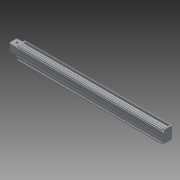
# Autodesk Inventor part: GL20N41420CSW' Body2
Saved by Autodesk Inventor 2011 SP1 (Build 150282100, 282)
## iProperties
Created: 2013-11-12
Part Number: GL20N41420CSW' Body2
Catalog Web Link: www.cadenas.de
Description: Type GL-N-body2-
Vendor: THK
Document SubType Name: Modeling
Designer: PARTuser1
Manufacturer: THK
Density: 1 g/cm^3
Category: PARTsolutions
Company: THK
Title: GL20N41420CSW' Body2
Author: Cadenas PARTsolutions
PSOL_IDENT_0: {$CADENAS_DATA\23d-libs\thk\actuator\type_gl_n\type_gl_n_f_na_1.prj},213 {VTYP=3D},{NB=GL20N41420CSW
PSOL_IDENT_1: ' Body2},{LINA=GL20N41420CSW' Body2},{NN=Type GL-N-body2},{DATE=29.11.2012 11:43:39},{GEOMDATE=29.11
PSOL_IDENT_2: .2012 11:43:00},{VERSION=},{LINEID=40},{LINESUBID=-1},{WBVAR=L,C,LM,BSE,BSM,LML,BSL}  {NB=GL20N41420
PSOL_IDENT_3: CSW' Body2},{LINA=GL20N41420CSW' Body2},{KT=DUMMY},{IDNR=},{MN=GL20N},{L=1420},{C=C},{LX=460,580,700
PSOL_IDENT_4: ,820,1060,1240,1420,1600,1780,1960,2200,2320,2500,3000},{LM=SW},{VER=4},{DS=Belt kit},{BSE=},{R=25.0
PSOL_IDENT_5: 00},{NDM=2.000},{PCD=0.000},{BSM=},{BSE1='','None'},{SD=39},{SD1=27},{TL=180.000},{B=65.000},{TL1=21
PSOL_IDENT_6: 0.000},{B1=70.000},{DS1=Ex},{LML='},{BSL=},{BSL1='','None'},{N=9},{N1=6},{N2=8.000},{N3=6},{BSM1='',
PSOL_IDENT_7: 'None'}
CNS_NN: Type GL-N-body2
CNS_NB: GL20N41420CSW' Body2
CNS_NBSYN: $MN.$VER.$L.$C.$BSE.$BSM.$LM.$LML.$BSL. Body2
CNS_LINA: GL20N41420CSW' Body2
CNS_MN: GL20N
CNS_L: 1420
CNS_C: Yes
CNS_LX: 460,580,700,820,1060,1240,1420,1600,1780,1960,2200,2320,2500,3000
CNS_LM: SSR-XW (L-type table)
CNS_VER: 4
CNS_DS: Belt kit
CNS_R: 25.000
CNS_NDM: 2.000
CNS_PCD: 0.000
CNS_BSE1: '','None'
CNS_SD: 39
CNS_SD1: 27
CNS_TL: 180.000
CNS_B: 65.000
CNS_TL1: 210.000
CNS_B1: 70.000
CNS_DS1: Ex
CNS_LML: No mark:Not provided with QZ
CNS_BSL1: '','None'
CNS_N: 9.000
CNS_N1: 6.000
CNS_N2: 8.000
CNS_N3: 6.000
CNS_BSM1: '','None'
SUPPLIER: THK
ARTICLENO: GL20N41420CSW' Body2
BOMINFO: GL20N41420CSW' Body2
CREATOR: CADENAS GmbH
Autodesk Inventor part; units mm, degrees
sketch "Sketch_1" plane through (0, 0, 0) normal (1, 0, 0) x (0, 1, 0)
  line L0 (39, 65) -> (37, 65)
  line L1 (37, 65) -> (37, 64)
  line L2 (37, 64) -> (33.72, 64)
  arc A0 (33.72, 64) -> (33.25, 63.53) centre (33.72, 63.53) ccw
  line L3 (33.25, 63.53) -> (33.25, 62.97)
  arc A1 (33.25, 62.97) -> (33.72, 62.5) centre (33.72, 62.97) ccw
  line L4 (33.72, 62.5) -> (33.93, 62.5)
  arc A2 (34.4, 62.03) -> (33.93, 62.5) centre (33.93, 62.03) ccw
  line L5 (34.4, 62.03) -> (34.4, 60.47)
  arc A3 (33.93, 60) -> (34.4, 60.47) centre (33.93, 60.47) ccw
  line L6 (33.93, 60) -> (33.7, 60)
  arc A4 (33.7, 60) -> (33.5, 59.8) centre (33.7, 59.8) ccw
  line L7 (33.5, 59.8) -> (33.5, 59.7)
  arc A5 (33.3, 59.5) -> (33.5, 59.7) centre (33.3, 59.7) ccw
  line L8 (33.3, 59.5) -> (29.7, 59.5)
  arc A6 (29.5, 59.7) -> (29.7, 59.5) centre (29.7, 59.7) ccw
  line L9 (29.5, 59.7) -> (29.5, 59.8)
  arc A7 (29.5, 59.8) -> (29.3, 60) centre (29.3, 59.8) ccw
  line L10 (29.3, 60) -> (29.07, 60)
  arc A8 (28.6, 60.47) -> (29.07, 60) centre (29.07, 60.47) ccw
  line L11 (28.6, 60.47) -> (28.6, 62.03)
  arc A9 (29.07, 62.5) -> (28.6, 62.03) centre (29.07, 62.03) ccw
  line L12 (29.07, 62.5) -> (29.28, 62.5)
  arc A10 (29.28, 62.5) -> (29.75, 62.97) centre (29.28, 62.97) ccw
  line L13 (29.75, 62.97) -> (29.75, 63.7)
  arc A11 (29.75, 63.7) -> (29.45, 64) centre (29.45, 63.7) ccw
  line L14 (29.45, 64) -> (26, 64)
  line L15 (26, 64) -> (26, 65)
  line L16 (26, 65) -> (12.3, 65)
  arc A12 (12.3, 65) -> (12, 64.7) centre (12.3, 64.7) ccw
  line L17 (12, 64.7) -> (12, 60.8)
  arc A13 (11.7, 60.5) -> (12, 60.8) centre (11.7, 60.8) ccw
  line L18 (11.7, 60.5) -> (6.3, 60.5)
  arc A14 (6, 60.8) -> (6.3, 60.5) centre (6.3, 60.8) ccw
  line L19 (6, 60.8) -> (6, 64.7)
  arc A15 (6, 64.7) -> (5.7, 65) centre (5.7, 64.7) ccw
  line L20 (5.7, 65) -> (3.14, 65)
  arc A16 (3.14, 65) -> (0, 61.86) centre (3.14, 61.86) ccw
  line L21 (0, 61.86) -> (0, 53.47)
  arc A17 (0, 53.47) -> (0.47, 53) centre (0.47, 53.47) ccw
  line L22 (0.47, 53) -> (3.53, 53)
  arc A18 (3.53, 53) -> (4, 53.47) centre (3.53, 53.47) ccw
  line L23 (4, 53.47) -> (4, 55.03)
  arc A19 (4.47, 55.5) -> (4, 55.03) centre (4.47, 55.03) ccw
  line L24 (4.47, 55.5) -> (8.53, 55.5)
  arc A20 (9, 55.03) -> (8.53, 55.5) centre (8.53, 55.03) ccw
  line L25 (9, 55.03) -> (9, 53.7)
  arc A21 (9, 53.7) -> (9.2, 53.5) centre (9.2, 53.7) ccw
  line L26 (9.2, 53.5) -> (9.53, 53.5)
  arc A22 (10, 53.03) -> (9.53, 53.5) centre (9.53, 53.03) ccw
  line L27 (10, 53.03) -> (10, 46.97)
  arc A23 (9.53, 46.5) -> (10, 46.97) centre (9.53, 46.97) ccw
  line L28 (9.53, 46.5) -> (9.2, 46.5)
  arc A24 (9.2, 46.5) -> (9, 46.3) centre (9.2, 46.3) ccw
  line L29 (9, 46.3) -> (9, 44.97)
  arc A25 (8.53, 44.5) -> (9, 44.97) centre (8.53, 44.97) ccw
  line L30 (8.53, 44.5) -> (4.47, 44.5)
  arc A26 (4, 44.97) -> (4.47, 44.5) centre (4.47, 44.97) ccw
  line L31 (4, 44.97) -> (4, 46.53)
  arc A27 (4, 46.53) -> (3.53, 47) centre (3.53, 46.53) ccw
  line L32 (3.53, 47) -> (0.47, 47)
  arc A28 (0.47, 47) -> (0, 46.53) centre (0.47, 46.53) ccw
  line L33 (0, 46.53) -> (0, 25)
  line L34 (0, 25) -> (1.3137, 18.3899)
  arc A29 (1.3469, 17.8569) -> (1.3137, 18.3899) centre (-0.6479, 18) ccw
  arc A30 (1.3469, 17.8569) -> (1.3469, -17.8569) centre (250.2071, 0) ccw
  arc A31 (1.3137, -18.3899) -> (1.3469, -17.8569) centre (-0.6479, -18) ccw
  line L35 (1.3137, -18.3899) -> (0, -25)
  line L36 (0, -25) -> (0, -46.53)
  arc A32 (0, -46.53) -> (0.47, -47) centre (0.47, -46.53) ccw
  line L37 (0.47, -47) -> (3.53, -47)
  arc A33 (3.53, -47) -> (4, -46.53) centre (3.53, -46.53) ccw
  line L38 (4, -46.53) -> (4, -44.97)
  arc A34 (4.47, -44.5) -> (4, -44.97) centre (4.47, -44.97) ccw
  line L39 (4.47, -44.5) -> (8.53, -44.5)
  arc A35 (9, -44.97) -> (8.53, -44.5) centre (8.53, -44.97) ccw
  line L40 (9, -44.97) -> (9, -46.3)
  arc A36 (9, -46.3) -> (9.2, -46.5) centre (9.2, -46.3) ccw
  line L41 (9.2, -46.5) -> (9.53, -46.5)
  arc A37 (10, -46.97) -> (9.53, -46.5) centre (9.53, -46.97) ccw
  line L42 (10, -46.97) -> (10, -53.03)
  arc A38 (9.53, -53.5) -> (10, -53.03) centre (9.53, -53.03) ccw
  line L43 (9.53, -53.5) -> (9.2, -53.5)
  arc A39 (9.2, -53.5) -> (9, -53.7) centre (9.2, -53.7) ccw
  line L44 (9, -53.7) -> (9, -55.03)
  arc A40 (8.53, -55.5) -> (9, -55.03) centre (8.53, -55.03) ccw
  line L45 (8.53, -55.5) -> (4.47, -55.5)
  arc A41 (4, -55.03) -> (4.47, -55.5) centre (4.47, -55.03) ccw
  line L46 (4, -55.03) -> (4, -53.47)
  arc A42 (4, -53.47) -> (3.53, -53) centre (3.53, -53.47) ccw
  line L47 (3.53, -53) -> (0.47, -53)
  arc A43 (0.47, -53) -> (0, -53.47) centre (0.47, -53.47) ccw
  line L48 (0, -53.47) -> (0, -61.86)
  arc A44 (0, -61.86) -> (3.14, -65) centre (3.14, -61.86) ccw
  line L49 (3.14, -65) -> (5.7, -65)
  arc A45 (5.7, -65) -> (6, -64.7) centre (5.7, -64.7) ccw
  line L50 (6, -64.7) -> (6, -60.8)
  arc A46 (6.3, -60.5) -> (6, -60.8) centre (6.3, -60.8) ccw
  line L51 (6.3, -60.5) -> (11.7, -60.5)
  arc A47 (12, -60.8) -> (11.7, -60.5) centre (11.7, -60.8) ccw
  line L52 (12, -60.8) -> (12, -64.7)
  arc A48 (12, -64.7) -> (12.3, -65) centre (12.3, -64.7) ccw
  line L53 (12.3, -65) -> (26, -65)
  line L54 (26, -65) -> (26, -64)
  line L55 (26, -64) -> (29.45, -64)
  arc A49 (29.45, -64) -> (29.75, -63.7) centre (29.45, -63.7) ccw
  line L56 (29.75, -63.7) -> (29.75, -62.97)
  arc A50 (29.75, -62.97) -> (29.28, -62.5) centre (29.28, -62.97) ccw
  line L57 (29.28, -62.5) -> (29.07, -62.5)
  arc A51 (28.6, -62.03) -> (29.07, -62.5) centre (29.07, -62.03) ccw
  line L58 (28.6, -62.03) -> (28.6, -60.47)
  arc A52 (29.07, -60) -> (28.6, -60.47) centre (29.07, -60.47) ccw
  line L59 (29.07, -60) -> (29.3, -60)
  arc A53 (29.3, -60) -> (29.5, -59.8) centre (29.3, -59.8) ccw
  line L60 (29.5, -59.8) -> (29.5, -59.7)
  arc A54 (29.7, -59.5) -> (29.5, -59.7) centre (29.7, -59.7) ccw
  line L61 (29.7, -59.5) -> (33.3, -59.5)
  arc A55 (33.5, -59.7) -> (33.3, -59.5) centre (33.3, -59.7) ccw
  line L62 (33.5, -59.7) -> (33.5, -59.8)
  arc A56 (33.5, -59.8) -> (33.7, -60) centre (33.7, -59.8) ccw
  line L63 (33.7, -60) -> (33.93, -60)
  arc A57 (34.4, -60.47) -> (33.93, -60) centre (33.93, -60.47) ccw
  line L64 (34.4, -60.47) -> (34.4, -62.03)
  arc A58 (33.93, -62.5) -> (34.4, -62.03) centre (33.93, -62.03) ccw
  line L65 (33.93, -62.5) -> (33.72, -62.5)
  arc A59 (33.72, -62.5) -> (33.25, -62.97) centre (33.72, -62.97) ccw
  line L66 (33.25, -62.97) -> (33.25, -63.53)
  arc A60 (33.25, -63.53) -> (33.72, -64) centre (33.72, -63.53) ccw
  line L67 (33.72, -64) -> (37, -64)
  line L68 (37, -64) -> (37, -65)
  line L69 (37, -65) -> (39, -65)
  line L70 (39, -65) -> (39, -41)
  line L71 (39, -41) -> (43.5, -41)
  line L72 (43.5, -41) -> (43.5, -37)
  line L73 (43.5, -37) -> (21, -37)
  arc A61 (19, -35) -> (21, -37) centre (21, -35) ccw
  line L74 (19, -35) -> (19, 35)
  arc A62 (21, 37) -> (19, 35) centre (21, 35) ccw
  line L75 (21, 37) -> (43.5, 37)
  line L76 (43.5, 37) -> (43.5, 41)
  line L77 (43.5, 41) -> (39, 41)
  line L78 (39, 41) -> (39, 65)
  constraints: 158 end point, 126 point on circle, 63 centre point
extrude "Extrusion1" add sketch "Sketch_1" along normal blind 1420
sketch "Sketch_41" plane through (0, 0, 0) normal (1, 0, 0) x (0, 1, 0)
  line L0 (54.4, -41) -> (51.5, -41)
  line L1 (51.5, -41) -> (49.5, -43)
  line L2 (49.5, -43) -> (46, -43)
  line L3 (46, -43) -> (44, -41)
  line L4 (44, -41) -> (40, -41)
  line L5 (40, -41) -> (39, -42)
  line L6 (39, -42) -> (39, -60)
  line L7 (39, -60) -> (40, -61)
  line L8 (40, -61) -> (44, -61)
  line L9 (44, -61) -> (46, -59)
  line L10 (46, -59) -> (49.5, -59)
  line L11 (49.5, -59) -> (51.5, -61)
  line L12 (51.5, -61) -> (54.4, -61)
  line L13 (54.4, -61) -> (55.5, -59.9)
  line L14 (55.5, -59.9) -> (55.5, -42.1)
  line L15 (55.5, -42.1) -> (54.4, -41)
  constraints: 32 end point
extrude "Extrusion2" add sketch "Sketch_41" along normal blind 1420
sketch "Sketch_42" plane through (0, 0, 0) normal (1, 0, 0) x (0, 1, 0)
  line L0 (51.5, 61) -> (49.5, 59)
  line L1 (49.5, 59) -> (46, 59)
  line L2 (46, 59) -> (44, 61)
  line L3 (44, 61) -> (40, 61)
  line L4 (40, 61) -> (39, 60)
  line L5 (39, 60) -> (39, 42)
  line L6 (39, 42) -> (40, 41)
  line L7 (40, 41) -> (44, 41)
  line L8 (44, 41) -> (46, 43)
  line L9 (46, 43) -> (49.5, 43)
  line L10 (49.5, 43) -> (51.5, 41)
  line L11 (51.5, 41) -> (54.4, 41)
  line L12 (54.4, 41) -> (55.5, 42.1)
  line L13 (55.5, 42.1) -> (55.5, 59.9)
  line L14 (55.5, 59.9) -> (54.4, 61)
  line L15 (54.4, 61) -> (51.5, 61)
  constraints: 32 end point
extrude "Extrusion3" add sketch "Sketch_42" along normal blind 1420
sketch "Sketch_2" plane through (0, 0, 0) normal (1, 0, 0) x (0, 1, 0)
  line L0 (82, 60) -> (13, 60)
  line L1 (13, 60) -> (11, 58)
  line L2 (11, 58) -> (11, 45.64)
  arc A0 (7.86, 42.5) -> (11, 45.64) centre (7.86, 45.64) ccw
  line L3 (7.86, 42.5) -> (4, 42.5)
  line L4 (4, 42.5) -> (2, 40.5)
  line L5 (2, 40.5) -> (2, -40.5)
  line L6 (2, -40.5) -> (4, -42.5)
  line L7 (4, -42.5) -> (7.86, -42.5)
  arc A1 (11, -45.64) -> (7.86, -42.5) centre (7.86, -45.64) ccw
  line L8 (11, -45.64) -> (11, -58)
  line L9 (11, -58) -> (13, -60)
  line L10 (13, -60) -> (82, -60)
  line L11 (82, -60) -> (83, -59)
  line L12 (83, -59) -> (83, -50)
  line L13 (83, -50) -> (87, -50)
  line L14 (87, -50) -> (87, 50)
  line L15 (87, 50) -> (83, 50)
  line L16 (83, 50) -> (83, 59)
  line L17 (83, 59) -> (82, 60)
  constraints: 36 end point, 4 point on circle, 2 centre point
extrude "Extrusion4" add sketch "Sketch_2" against normal blind 12
sketch "Sketch_3" plane through (1420, 0, 0) normal (1, 0, 0) x (0, 0, -1)
  line L0 (-60, 82) -> (-60, 13)
  line L1 (-60, 13) -> (-58, 11)
  line L2 (-58, 11) -> (-45.64, 11)
  arc A0 (-42.5, 7.86) -> (-45.64, 11) centre (-45.64, 7.86) ccw
  line L3 (-42.5, 7.86) -> (-42.5, 4)
  line L4 (-42.5, 4) -> (-40.5, 2)
  line L5 (-40.5, 2) -> (40.5, 2)
  line L6 (40.5, 2) -> (42.5, 4)
  line L7 (42.5, 4) -> (42.5, 7.86)
  arc A1 (45.64, 11) -> (42.5, 7.86) centre (45.64, 7.86) ccw
  line L8 (45.64, 11) -> (58, 11)
  line L9 (58, 11) -> (60, 13)
  line L10 (60, 13) -> (60, 82)
  line L11 (60, 82) -> (59, 83)
  line L12 (59, 83) -> (50, 83)
  line L13 (50, 83) -> (50, 87)
  line L14 (50, 87) -> (-50, 87)
  line L15 (-50, 87) -> (-50, 83)
  line L16 (-50, 83) -> (-59, 83)
  line L17 (-59, 83) -> (-60, 82)
  constraints: 36 end point, 4 point on circle, 2 centre point
extrude "Extrusion5" add sketch "Sketch_3" along normal blind 12
sketch "Sketch_5" plane through (0, 0, 0) normal (1, 0, 0) x (0, 1, 0)
  line L0 (80.8094, -15) -> (76.1906, -15)
  line L1 (76.1906, -15) -> (73.8812, -19)
  line L2 (73.8812, -19) -> (76.1906, -23)
  line L3 (76.1906, -23) -> (80.8094, -23)
  line L4 (80.8094, -23) -> (83.1188, -19)
  line L5 (83.1188, -19) -> (80.8094, -15)
  constraints: 12 end point
extrude "Extrusion6" add sketch "Sketch_5" along normal blind 3.2
sketch "Sketch_6" plane through (0, 0, -19) normal (0, 0, 1) x (1, 0, 0)
  line L0 (15, 78.5) -> (3.2, 78.5)
  line L1 (3.2, 78.5) -> (3.2, 81)
  line L2 (3.2, 81) -> (6, 81)
  line L3 (6, 81) -> (6, 84.75)
  line L4 (6, 84.75) -> (15, 84.75)
  line L5 (15, 84.75) -> (15, 78.5)
  line L6 (15, 78.5) -> (3.2, 78.5)
  constraints: 14 end point
revolve "Revolution1" add sketch "Sketch_6" angle 360 about axis through (15, 78.5, -19) along (1, 0, 0)
sketch "Sketch8" plane through (1432, 0, 0) normal (1, 0, 0) x (0, 0, -1)
  point P0 (0, 78.5)
hole "Drilling 1" at (1432, 78.5, 0) direction (-1, 0, 0) diameter 4.134 depth 12 countersink diameter 5 countersink angle 90 thread size "M5x0.8" class "6H" standard "ISO Metric profile"
sketch "Sketch_7" plane through (1417.5, 0, 0) normal (1, 0, 0) x (0, 0, -1)
  line L0 (-29, 19) -> (29, 19)
  line L1 (29, 19) -> (29, 40.5)
  line L2 (29, 40.5) -> (-29, 40.5)
  line L3 (-29, 40.5) -> (-29, 19)
  constraints: 8 end point
extrude "Extrusion7" add sketch "Sketch_7" against normal blind 63
sketch "Sketch_8" plane through (0, 40.5, 0) normal (0, 1, 0) x (1, 0, 0)
  line L0 (1322, -29) -> (1403, -29)
  line L1 (1403, -29) -> (1403, 29)
  line L2 (1403, 29) -> (1322, 29)
  line L3 (1322, 29) -> (1322, 17)
  line L4 (1322, 17) -> (1357, 17)
  line L5 (1357, 17) -> (1357, -17)
  line L6 (1357, -17) -> (1322, -17)
  line L7 (1322, -17) -> (1322, -29)
  arc A0 (1362, -20.4) -> (1362, -25.6) centre (1362, -23) ccw
  line L8 (1362, -25.6) -> (1396, -25.6)
  arc A1 (1396, -25.6) -> (1396, -20.4) centre (1396, -23) ccw
  line L9 (1396, -20.4) -> (1362, -20.4)
  arc A2 (1362, 25.6) -> (1362, 20.4) centre (1362, 23) ccw
  line L10 (1362, 20.4) -> (1396, 20.4)
  arc A3 (1396, 20.4) -> (1396, 25.6) centre (1396, 23) ccw
  line L11 (1396, 25.6) -> (1362, 25.6)
  constraints: 24 end point, 8 point on circle, 4 centre point
extrude "Extrusion8" add sketch "Sketch_8" along normal blind 20
sketch "Sketch_9" plane through (0, 0, 0) normal (0, 0, 1) x (1, 0, 0)
  line L0 (-92, 84.3) -> (-92, 16.7)
  line L1 (-92, 16.7) -> (-87.8, 12.5)
  line L2 (-87.8, 12.5) -> (-12, 12.5)
  line L3 (-12, 12.5) -> (-12, 88.5)
  line L4 (-12, 88.5) -> (-87.8, 88.5)
  line L5 (-87.8, 88.5) -> (-92, 84.3)
  constraints: 12 end point
extrude "Extrusion9" add sketch "Sketch_9" along normal mid plane 72
sketch "Sketch_14" plane through (0, 25.5, 0) normal (0, 1, 0) x (1, 0, 0)
  arc A0 (-57, 25) -> (-57, -25) centre (-57, 0) ccw
  line L0 (-57, -25) -> (-12, -25)
  line L1 (-12, -25) -> (-12, -26)
  line L2 (-12, -26) -> (0, -26)
  line L3 (0, -26) -> (0, 24)
  line L4 (0, 24) -> (-12, 24)
  line L5 (-12, 24) -> (-12, 25)
  line L6 (-12, 25) -> (-57, 25)
  constraints: 14 end point, 2 point on circle, 1 centre point
extrude "Extrusion10" cut sketch "Sketch_14" along normal blind 50
sketch "Sketch_15" plane through (1332, 0, 0) normal (1, 0, 0) x (0, 0, -1)
  line L0 (31.15, 50.5) -> (-31.15, 50.5)
  line L1 (-31.15, 50.5) -> (-31.15, 55.5)
  line L2 (-31.15, 55.5) -> (-15.75, 55.5)
  line L3 (-15.75, 55.5) -> (-15.75, 66)
  line L4 (-15.75, 66) -> (-15.3, 66)
  line L5 (-15.3, 66) -> (-15.3, 73)
  line L6 (-15.3, 73) -> (-13.8, 73)
  line L7 (-13.8, 73) -> (-13.3, 69)
  line L8 (-13.3, 69) -> (13.3, 69)
  line L9 (13.3, 69) -> (13.8, 73)
  line L10 (13.8, 73) -> (15.3, 73)
  line L11 (15.3, 73) -> (15.3, 66)
  line L12 (15.3, 66) -> (15.75, 66)
  line L13 (15.75, 66) -> (15.75, 55.5)
  line L14 (15.75, 55.5) -> (31.15, 55.5)
  line L15 (31.15, 55.5) -> (31.15, 50.5)
  line L16 (31.15, 50.5) -> (-31.15, 50.5)
  constraints: 34 end point
revolve "Revolution2" add sketch "Sketch_15" angle 360 about axis through (1332, 50.5, -31.15) along (0, 0, -1)
sketch "Sketch14" plane through (0, 0, 36) normal (0, 0, 1) x (1, 0, 0)
  point P0 (-52, 50.5)
hole "Drilling 2" at (-52, 50.5, 36) direction (0, 0, -1) diameter 22 depth 4
sketch "Sketch15" plane through (0, 0, -36) normal (0, 0, -1) x (-1, 0, 0)
  point P0 (52, 50.5)
hole "Drilling 3" at (-52, 50.5, -36) direction (0, 0, 1) diameter 22 depth 4
sketch "Sketch_18" plane through (-52, 0, 0) normal (1, 0, 0) x (0, 0, -1)
  line L0 (35.55, 50.5) -> (-51, 50.5)
  line L1 (-51, 50.5) -> (-51, 56)
  line L2 (-51, 56) -> (-50.5, 56.5)
  line L3 (-50.5, 56.5) -> (-15.75, 56.5)
  line L4 (-15.75, 56.5) -> (-15.75, 66)
  line L5 (-15.75, 66) -> (-15.3, 66)
  line L6 (-15.3, 66) -> (-15.3, 73)
  line L7 (-15.3, 73) -> (-13.8, 73)
  line L8 (-13.8, 73) -> (-13.3, 69)
  line L9 (-13.3, 69) -> (13.3, 69)
  line L10 (13.3, 69) -> (13.8, 73)
  line L11 (13.8, 73) -> (15.3, 73)
  line L12 (15.3, 73) -> (15.3, 66)
  line L13 (15.3, 66) -> (15.75, 66)
  line L14 (15.75, 66) -> (15.75, 56.5)
  line L15 (15.75, 56.5) -> (35.55, 56.5)
  line L16 (35.55, 56.5) -> (35.55, 50.5)
  line L17 (35.55, 50.5) -> (-51, 50.5)
  constraints: 36 end point
revolve "Revolution3" add sketch "Sketch_18" angle 360 about axis through (-52, 50.5, -35.55) along (0, 0, -1)
sketch "Sketch_19" plane through (0, 0, 0) normal (0, 0, 1) x (1, 0, 0)
  arc A0 (-54.95, 69.95) -> (-54.95, 31.05) centre (-54.95, 50.5) ccw
  line L0 (-54.95, 31.05) -> (1331.5, 31.05)
  arc A1 (1331.5, 31.05) -> (1331.5, 69.95) centre (1331.5, 50.5) ccw
  line L1 (1331.5, 69.95) -> (-54.95, 69.95)
  arc A2 (-54.95, 67) -> (-54.95, 34) centre (-54.95, 50.5) ccw
  line L2 (-54.95, 34) -> (1331.5, 34)
  arc A3 (1331.5, 34) -> (1331.5, 67) centre (1331.5, 50.5) ccw
  line L3 (1331.5, 67) -> (-54.95, 67)
  constraints: 8 end point, 8 point on circle, 4 centre point
extrude "Extrusion11" add sketch "Sketch_19" along normal mid plane 25
sketch "Sketch_20" plane through (1409.5, 0, 0) normal (1, 0, 0) x (0, 0, -1)
  line L0 (23, 40.5) -> (23, 47.5)
  line L1 (23, 47.5) -> (28, 47.5)
  line L2 (28, 47.5) -> (28, 41.5)
  line L3 (28, 41.5) -> (28.5, 41.5)
  line L4 (28.5, 41.5) -> (28.5, 40.5)
  line L5 (28.5, 40.5) -> (23, 40.5)
  line L6 (23, 40.5) -> (23, 47.5)
  constraints: 14 end point
revolve "Revolution4" add sketch "Sketch_20" angle 360 about axis through (1409.5, 40.5, -23) along (0, -1, 0)
sketch "Sketch_21" plane through (1409.5, 0, 0) normal (1, 0, 0) x (0, 0, -1)
  line L0 (-23, 40.5) -> (-23, 47.5)
  line L1 (-23, 47.5) -> (-18, 47.5)
  line L2 (-18, 47.5) -> (-18, 41.5)
  line L3 (-18, 41.5) -> (-17.5, 41.5)
  line L4 (-17.5, 41.5) -> (-17.5, 40.5)
  line L5 (-17.5, 40.5) -> (-23, 40.5)
  line L6 (-23, 40.5) -> (-23, 47.5)
  constraints: 14 end point
revolve "Revolution5" add sketch "Sketch_21" angle 360 about axis through (1409.5, 40.5, 23) along (0, -1, 0)
sketch "Sketch_22" plane through (1396, 0, 0) normal (1, 0, 0) x (0, 0, -1)
  line L0 (23, 60.5) -> (23, 66.5)
  line L1 (23, 66.5) -> (27.25, 66.5)
  line L2 (27.25, 66.5) -> (27.25, 61.5)
  line L3 (27.25, 61.5) -> (28, 61.5)
  line L4 (28, 61.5) -> (28, 60.5)
  line L5 (28, 60.5) -> (23, 60.5)
  line L6 (23, 60.5) -> (23, 66.5)
  constraints: 14 end point
revolve "Revolution6" add sketch "Sketch_22" angle 360 about axis through (1396, 60.5, -23) along (0, -1, 0)
sketch "Sketch_23" plane through (1396, 0, 0) normal (1, 0, 0) x (0, 0, -1)
  line L0 (-23, 60.5) -> (-23, 66.5)
  line L1 (-23, 66.5) -> (-18.75, 66.5)
  line L2 (-18.75, 66.5) -> (-18.75, 61.5)
  line L3 (-18.75, 61.5) -> (-18, 61.5)
  line L4 (-18, 61.5) -> (-18, 60.5)
  line L5 (-18, 60.5) -> (-23, 60.5)
  line L6 (-23, 60.5) -> (-23, 66.5)
  constraints: 14 end point
revolve "Revolution7" add sketch "Sketch_23" angle 360 about axis through (1396, 60.5, 23) along (0, -1, 0)
sketch "Sketch_24" plane through (1376, 0, 0) normal (1, 0, 0) x (0, 0, -1)
  line L0 (23, 60.5) -> (23, 66.5)
  line L1 (23, 66.5) -> (27.25, 66.5)
  line L2 (27.25, 66.5) -> (27.25, 61.5)
  line L3 (27.25, 61.5) -> (28, 61.5)
  line L4 (28, 61.5) -> (28, 60.5)
  line L5 (28, 60.5) -> (23, 60.5)
  line L6 (23, 60.5) -> (23, 66.5)
  constraints: 14 end point
revolve "Revolution8" add sketch "Sketch_24" angle 360 about axis through (1376, 60.5, -23) along (0, -1, 0)
sketch "Sketch_25" plane through (1376, 0, 0) normal (1, 0, 0) x (0, 0, -1)
  line L0 (-23, 60.5) -> (-23, 66.5)
  line L1 (-23, 66.5) -> (-18.75, 66.5)
  line L2 (-18.75, 66.5) -> (-18.75, 61.5)
  line L3 (-18.75, 61.5) -> (-18, 61.5)
  line L4 (-18, 61.5) -> (-18, 60.5)
  line L5 (-18, 60.5) -> (-23, 60.5)
  line L6 (-23, 60.5) -> (-23, 66.5)
  constraints: 14 end point
revolve "Revolution9" add sketch "Sketch_25" angle 360 about axis through (1376, 60.5, 23) along (0, -1, 0)
sketch "Sketch24" plane through (0, 0, 36) normal (0, 0, 1) x (1, 0, 0)
  point P0 (-78.87, 77.37)
hole "Drilling 4" at (-78.87, 77.37, 36) direction (0, 0, -1) diameter 4.134 depth 9.6 tip angle 119.725 countersink diameter 5 countersink angle 90 thread size "M5x0.8" class "6H" standard "ISO Metric profile"
sketch "Sketch25" plane through (0, 0, 36) normal (0, 0, 1) x (1, 0, 0)
  point P0 (-78.87, 23.63)
hole "Drilling 5" at (-78.87, 23.63, 36) direction (0, 0, -1) diameter 4.134 depth 9.6 tip angle 119.725 countersink diameter 5 countersink angle 90 thread size "M5x0.8" class "6H" standard "ISO Metric profile"
sketch "Sketch26" plane through (0, 0, 36) normal (0, 0, 1) x (1, 0, 0)
  point P0 (-25.13, 77.37)
hole "Drilling 6" at (-25.13, 77.37, 36) direction (0, 0, -1) diameter 4.134 depth 9.6 tip angle 119.725 countersink diameter 5 countersink angle 90 thread size "M5x0.8" class "6H" standard "ISO Metric profile"
sketch "Sketch27" plane through (0, 0, 36) normal (0, 0, 1) x (1, 0, 0)
  point P0 (-25.13, 23.63)
hole "Drilling 7" at (-25.13, 23.63, 36) direction (0, 0, -1) diameter 4.134 depth 9.6 tip angle 119.725 countersink diameter 5 countersink angle 90 thread size "M5x0.8" class "6H" standard "ISO Metric profile"
sketch "Sketch_30" plane through (-12, 0, 0) normal (1, 0, 0) x (0, 0, -1)
  line L0 (-59, 87.24) -> (-59, 84.26)
  arc A0 (-59, 84.26) -> (-57.74, 83) centre (-57.74, 84.26) ccw
  line L1 (-57.74, 83) -> (-51, 83)
  line L2 (-51, 83) -> (-51, 84.5)
  line L3 (-51, 84.5) -> (-57.5, 84.5)
  line L4 (-57.5, 84.5) -> (-57.5, 87)
  line L5 (-57.5, 87) -> (57.5, 87)
  line L6 (57.5, 87) -> (57.5, 84.5)
  line L7 (57.5, 84.5) -> (51, 84.5)
  line L8 (51, 84.5) -> (51, 83)
  line L9 (51, 83) -> (57.74, 83)
  arc A1 (57.74, 83) -> (59, 84.26) centre (57.74, 84.26) ccw
  line L10 (59, 84.26) -> (59, 87.24)
  arc A2 (59, 87.24) -> (57.74, 88.5) centre (57.74, 87.24) ccw
  line L11 (57.74, 88.5) -> (-57.74, 88.5)
  arc A3 (-57.74, 88.5) -> (-59, 87.24) centre (-57.74, 87.24) ccw
  constraints: 24 end point, 8 point on circle, 4 centre point
extrude "Extrusion12" add sketch "Sketch_30" along normal blind 1444
sketch "Sketch_31" plane through (0, 0, -32) normal (0, 0, 1) x (1, 0, 0)
  line L0 (-6, 88.5) -> (-6, 89.7)
  line L1 (-6, 89.7) -> (-2, 89.7)
  line L2 (-2, 89.7) -> (-2, 88.5)
  line L3 (-2, 88.5) -> (-6, 88.5)
  line L4 (-6, 88.5) -> (-6, 89.7)
  constraints: 10 end point
revolve "Revolution10" add sketch "Sketch_31" angle 360 about axis through (-6, 88.5, -32) along (0, -1, 0)
sketch "Sketch_32" plane through (0, 0, 32) normal (0, 0, 1) x (1, 0, 0)
  line L0 (1426, 88.5) -> (1426, 89.7)
  line L1 (1426, 89.7) -> (1430, 89.7)
  line L2 (1430, 89.7) -> (1430, 88.5)
  line L3 (1430, 88.5) -> (1426, 88.5)
  line L4 (1426, 88.5) -> (1426, 89.7)
  constraints: 10 end point
revolve "Revolution11" add sketch "Sketch_32" angle 360 about axis through (1426, 88.5, 32) along (0, -1, 0)
sketch "Sketch_33" plane through (0, 0, -32) normal (0, 0, 1) x (1, 0, 0)
  line L0 (1426, 88.5) -> (1426, 89.7)
  line L1 (1426, 89.7) -> (1430, 89.7)
  line L2 (1430, 89.7) -> (1430, 88.5)
  line L3 (1430, 88.5) -> (1426, 88.5)
  line L4 (1426, 88.5) -> (1426, 89.7)
  constraints: 10 end point
revolve "Revolution12" add sketch "Sketch_33" angle 360 about axis through (1426, 88.5, -32) along (0, -1, 0)
sketch "Sketch_34" plane through (0, 0, 32) normal (0, 0, 1) x (1, 0, 0)
  line L0 (-6, 88.5) -> (-6, 89.7)
  line L1 (-6, 89.7) -> (-2, 89.7)
  line L2 (-2, 89.7) -> (-2, 88.5)
  line L3 (-2, 88.5) -> (-6, 88.5)
  line L4 (-6, 88.5) -> (-6, 89.7)
  constraints: 10 end point
revolve "Revolution13" add sketch "Sketch_34" angle 360 about axis through (-6, 88.5, 32) along (0, -1, 0)
sketch "Sketch33" plane through (0, 19, 35) normal (0, 1, 0) x (1, 0, 0)
  point P0 (80, 65)
hole "Drilling 8" at (80, 19, -30) direction (0, -1, 0) diameter 6.6 depth 19 counterbore diameter 11 counterbore depth 11
sketch "Sketch34" plane through (0, 19, 35) normal (0, 1, 0) x (1, 0, 0)
  point P0 (80, 5)
hole "Drilling 9" at (80, 19, 30) direction (0, -1, 0) diameter 6.6 depth 19 counterbore diameter 11 counterbore depth 11
pattern_linear "Rectangular Pattern1" count 7 spacing 200 along (1, 0, 0) of "Drilling 9"
pattern_linear "Rectangular Pattern2" count 7 spacing 200 along (1, 0, 0) of "Drilling 8"
ref_plane "type_gl_n_bt_XY" through (15, 44, 0) normal (-1, 0, 0) x (0, 0, -1)
ref_plane "type_gl_n_bt_YZ" through (15, 44, 0) normal (0, 0, -1) x (0, -1, 0)
ref_plane "type_gl_n_bt_ZX" through (15, 44, 0) normal (0, -1, 0) x (-1, 0, 0)
ref_plane "type_gl_n_bx_XY" through (-52, 50.5, 36) normal (0, 0, -1) x (1, 0, 0)
ref_plane "type_gl_n_bx_YZ" through (-52, 50.5, 36) normal (1, 0, 0) x (0, -1, 0)
ref_plane "type_gl_n_bx_ZX" through (-52, 50.5, 36) normal (0, -1, 0) x (0, 0, -1)
ref_plane "type_gl_n_dummy1_XY" through (0, 0, 0) normal (0, 1, 0) x (1, 0, 0)
ref_plane "type_gl_n_dummy1_YZ" through (0, 0, 0) normal (1, 0, 0) x (0, 0, -1)
ref_plane "type_gl_n_dummy1_ZX" through (0, 0, 0) normal (0, 0, -1) x (0, 1, 0)
ref_plane "type_gl_n_s1_XY" through (55.49, 31.6, 60) normal (0, 0, -1) x (1, 0, 0)
ref_plane "type_gl_n_s1_YZ" through (55.49, 31.6, 60) normal (1, 0, 0) x (0, -1, 0)
ref_plane "type_gl_n_s1_ZX" through (55.49, 31.6, 60) normal (0, -1, 0) x (0, 0, -1)
ref_plane "type_gl_n_s2_XY" through (627.995, 31.6, 60) normal (0, 0, -1) x (1, 0, 0)
ref_plane "type_gl_n_s2_YZ" through (627.995, 31.6, 60) normal (1, 0, 0) x (0, -1, 0)
ref_plane "type_gl_n_s2_ZX" through (627.995, 31.6, 60) normal (0, -1, 0) x (0, 0, -1)
ref_plane "type_gl_n_s3_XY" through (1200.5, 31.6, 60) normal (0, 0, -1) x (1, 0, 0)
ref_plane "type_gl_n_s3_YZ" through (1200.5, 31.6, 60) normal (1, 0, 0) x (0, -1, 0)
ref_plane "type_gl_n_s3_ZX" through (1200.5, 31.6, 60) normal (0, -1, 0) x (0, 0, -1)
body "Solid1"
